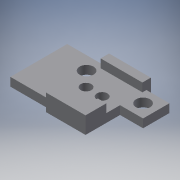
# Autodesk Inventor part: SensorMount
Saved by Autodesk Inventor 2018 (Build 220112000, 112)
## iProperties
Created: 2018-05-09
Part Number: SensorMount
Material: Generic
Document SubType Name: Modeling
Designer: s4321966
Mass: 0.644529 g
Surface Area: 8.91891 cm^2
Volume: 0.644529 cm^3
Density: 1 g/cm^3
Appearance: Default
Author: s4321966
Autodesk Inventor part; units mm, degrees
ref_plane "YZ Plane" through (0, 0, 0) normal (1, 0, 0) x (0, 1, 0)
ref_plane "XZ Plane" through (0, 0, 0) normal (0, 1, 0) x (-1, 0, 0)
ref_plane "XY Plane" through (0, 0, 0) normal (0, 0, 1) x (1, 0, 0)
sketch "Sketch1" plane through (0, 0, 0) normal (0, 0, 1) x (1, 0, 0)
  line L0 (0, 0) -> (15.75, 0)
  line L1 (15.75, 0) -> (15.75, -11.43)
  line L2 (15.75, -11.43) -> (0, -11.43)
  line L3 (0, -11.43) -> (0, 0)
  line L4 (17.75, 2) -> (-2, 2)
  line L5 (-2, 2) -> (-2, -13.43)
  line L6 (-2, -13.43) -> (17.75, -13.43)
  line L7 (17.75, -13.43) -> (17.75, 2)
  dimension "d0" = 15.75
  dimension "d1" = 11.43
  dimension "d2" = 2
  constraints: 16 end point, 4 parallel, 2 perpendicular, 1 horizontal, 3 other
  measures "d0" distance of L1.end L2.end
  measures "d1" distance of L0.end L1.end
  measures "d2" distance between parallel lines of L0 L4
extrude "Extrusion1" add sketch "Sketch1" along normal blind 2
sketch "Sketch2" plane through (0, 0, 0) normal (0, 0, -1) x (-1, 0, 0)
  line L0 (-17.75, 2) -> (2, 2) projected
  line L1 (2, -13.43) -> (-17.75, -13.43) projected
  line L2 (2, 2) -> (-17.75, 2)
  line L3 (-17.75, 2) -> (-17.75, -13.43)
  line L4 (-17.75, -13.43) -> (2, -13.43)
  line L5 (2, -13.43) -> (2, 2)
  point P0 (0, 0)
  constraints: 8 end point, 2 parallel, 1 horizontal, 1 perpendicular
extrude "Extrusion2" add sketch "Sketch2" along normal blind 2
sketch "Sketch3" plane through (0, 0, 0) normal (0, 0, 1) x (1, 0, 0)
  line L0 (0, 0) -> (15.75, 0) projected
  line L1 (0, 0) -> (6.73, 0)
  line L2 (0, 0) -> (6.73, 0) construction
  line L3 (6.73, 0) -> (6.73, -2.16)
  line L4 (15.75, 0) -> (13.84, 0)
  line L5 (15.75, 0) -> (17.66, 0) construction
  line L6 (13.84, 0) -> (13.84, -5.59)
  line L7 (13.84, -5.59) -> (10.04, -5.59)
  circle A0 centre (6.73, -2.16) radius 1.651
  circle A1 centre (10.04, -5.59) radius 1.25
  circle A2 centre (13.84, -5.59) radius 1.25
  dimension "d7" = 6.73
  dimension "d8" = 0
  dimension "d9" = 2.16
  dimension "d10" = 90
  dimension "d11" = 1.91
  dimension "d12" = 180
  dimension "d13" = 5.59
  dimension "d14" = 90
  dimension "d15" = 3.8
  dimension "d16" = 90
  dimension "d17" = 3.302
  dimension "d18" = 2.5
  dimension "d19" = 2.5
  constraints: 14 end point, 3 centre point, 3 coincident, 3 collinear, 3 horizontal, 3 perpendicular
  measures "d7" distance of L0.start L1.end
  measures "d8" distance between parallel lines of L1 L2
  measures "d9" distance of L1.end L3.end
  measures "d10" angle of L1 L3
  measures "d11" distance of L0.end L4.end
  measures "d12" angle of L4 L5
  measures "d13" distance of L4.end L6.end
  measures "d14" angle of L6 L4
  measures "d15" distance of L6.end L7.end
  measures "d16" angle of L6 L7
  measures "d17" diameter of A0
  measures "d18" diameter of A1
  measures "d19" diameter of A2
extrude "Extrusion3" cut sketch "Sketch3" against normal blind 2
sketch "Sketch4" plane through (0, 0, 0) normal (0, 0, 1) x (1, 0, 0)
  circle A0 centre (6.73, -2.16) radius 1.651 projected
  line L0 (6.73, -2.16) -> (-3.27, -2.16)
  circle A1 centre (-3.27, -2.16) radius 1.651
  line L1 (-2, 2) -> (17.75, 2) projected
  line L2 (7.875, 2) -> (-2, 2)
  line L3 (-2, 2) -> (-2, 0)
  line L4 (-2, 0) -> (7.875, 0)
  line L5 (7.875, 0) -> (7.875, 2)
  line L6 (0, -11.43) -> (15.75, -11.43) projected
  line L7 (-2, -13.43) -> (-2, 2) projected
  line L8 (8.381, -11.43) -> (-2, -11.43)
  line L9 (-2, -11.43) -> (-2, -13.43)
  line L10 (-2, -13.43) -> (8.381, -13.43)
  line L11 (8.381, -13.43) -> (8.381, -11.43)
  line L12 (15.75, 0) -> (0, 0) projected
  line L13 (0, 0) -> (-3.27, 0)
  line L14 (-3.27, 0) -> (-3.27, -0.509)
  line L15 (-3.27, -0.509) -> (0, -0.509)
  line L16 (0, -0.509) -> (0, 0)
  line L17 (0, 0) -> (-2, 0)
  line L18 (-2, 0) -> (-2, -11.43)
  line L19 (-2, -11.43) -> (0, -11.43)
  line L20 (0, -11.43) -> (0, 0)
  dimension "d23" = 3.302
  dimension "d22" = 10
  constraints: 34 end point, 8 parallel, 5 horizontal, 4 perpendicular, 1 coincident, 1 midpoint, 1 point on line, 1 vertical alignment, 2 other
  measures "d22" distance of L0.start L0.end
extrude "Extrusion4" cut sketch "Sketch4" along normal mid plane 4 contours L20 L8 L7 A1 L0 | L0 A1 L7 L15 L20 | A1 L7 L0 | L0 L7 A1 | L6 L11 L10 L7 L8 | L15 L7 L4 L16 | L7 A1 | L4 L3 L1 L5
sketch "Sketch5" plane through (0, 0, 0) normal (0, 0, 1) x (1, 0, 0)
  line L0 (15.7294, 0) -> (23.6467, -7.9173)
  line L1 (15.7294, 0) -> (26.9261, 0) construction
  circle A0 centre (13.84, -5.59) radius 1.25 projected
  line L2 (15.09, -5.59) -> (32.9108, -5.59)
  line L3 (32.9108, -5.59) -> (21.3194, -5.59)
  line L4 (21.3194, 0) -> (21.3194, -5.59)
  line L5 (21.3194, -2.795) -> (18.5244, -2.795)
  circle A1 centre (18.5244, -2.795) radius 1.651
  circle A2 centre (6.73, -2.16) radius 1.651 projected
  line L6 (6.73, -2.16) -> (27.3666, -2.16)
  line L7 (18.5244, -2.795) -> (18.5244, 1.4805)
  circle A3 centre (18.5244, -2.16) radius 1.65
  line L8 (17.75, 2) -> (17.75, -13.43) projected
  line L9 (21.3194, 0) -> (17.75, 0)
  line L10 (17.75, 0) -> (17.75, -5.59)
  line L11 (17.75, -5.59) -> (21.3194, -5.59)
  line L12 (21.3194, -5.59) -> (21.3194, 0)
  point P0 (0, 0)
  dimension "d26" = 45
  dimension "d27" = 3.302
  dimension "d28" = 3.3
  constraints: 24 end point, 9 point on line, 5 horizontal, 2 centre point, 2 parallel, 1 coincident, 1 equal length, 1 horizontal alignment, 1 midpoint, 1 perpendicular, 1 vertical, 1 other
  measures "d26" angle of L0 L1
  measures "d27" diameter of A1
  measures "d28" diameter of A3
extrude "Extrusion5" add sketch "Sketch5" against normal blind 2 contours L8 L9 L7 A3 | A3 L7 A1 L8 | L8 A1 L7 L6 L0 | L0 L6 L8 | A3 L6 A1 L7 | L7 L9 L4 L6 A3 | L6 L7 L0 | L0 A3 L8 L6 | A1 L6 L7 | A3 A1 L6 | L6 L4 L5 A1 A3 | L8 A3 L0 A1 | A1 L0 L2 L8 | L5 A3 L0 | L7 L6 A1 A3 L5 | A1 L5 A3 | A1 L5 L4 L0 | L0 A3 L5 A1 picked at (20.1034, -2.1943) picked at (18.7532, -3.9974)
sketch "Sketch6" plane through (0, 0, 2) normal (0, 0, 1) x (1, 0, 0)
  line L0 (21.3194, -5.59) -> (17.75, -5.59) projected
  line L1 (15.75, 0) -> (7.875, 0) projected
  line L2 (17.75, -5.59) -> (15.75, -5.59)
  line L3 (15.75, -5.59) -> (15.75, 0)
  line L4 (15.75, 0) -> (17.75, 0)
  line L5 (17.75, 0) -> (17.75, -5.59)
  line L6 (15.75, -5.59) -> (17.75, -5.59)
  line L7 (17.75, -5.59) -> (17.75, -11.43)
  line L8 (17.75, -11.43) -> (15.75, -11.43)
  line L9 (15.75, -11.43) -> (15.75, -5.59)
  line L10 (15.75, -11.43) -> (15.75, 0) projected
  line L11 (15.75, -8.51) -> (17.75, -8.51)
  line L12 (17.75, -8.51) -> (17.75, -11.43)
  line L13 (17.75, -11.43) -> (15.75, -11.43)
  line L14 (15.75, -11.43) -> (15.75, -8.51)
  point P0 (0, 0)
  constraints: 24 end point, 6 parallel, 3 horizontal, 3 perpendicular, 2 point on line
extrude "Extrusion6" cut sketch "Sketch6" against normal blind 2 contours L7 L11 L9 L2 | L2 L3 L4 L5
sketch "Sketch7" plane through (0, 0, 0) normal (0, 0, 1) x (1, 0, 0)
  circle A0 centre (6.73, -2.16) radius 1.651 projected
  line L0 (6.73, -2.16) -> (25.5258, -2.16)
  line L1 (6.7656, -0.5094) -> (22.9068, -0.5094)
  line L2 (21.3194, 0) -> (17.75, 0) projected
  circle A1 centre (21.3194, 0) radius 0.5094
  line L3 (20.81, 0) -> (20.81, -6.6139)
  line L4 (20.81, -0.5094) -> (15.4003, -5.9192)
  line L5 (20.81, -0.5094) -> (28.4606, -0.5094) construction
  circle A2 centre (19.1594, -2.16) radius 1.651
  point P0 (0, 0)
  dimension "d33" = 135
  dimension "d34" = 3.302
  constraints: 10 end point, 5 point on line, 3 horizontal, 1 centre point, 1 equal length, 1 horizontal alignment, 1 perpendicular, 1 vertical, 4 other
  measures "d33" angle of L4 L5
  measures "d34" diameter of A2
extrude "Extrusion7" cut sketch "Sketch7" against normal blind 2 contours A2 L4 L0 | L0 L4 A2 | L4 A2 L0 | L0 A2 L4
sketch "Sketch8" plane through (0, 0, 0) normal (0, 0, 1) x (1, 0, 0)
  line L0 (15.75, -11.43) -> (15.75, -8.51) projected
  line L1 (15.75, -8.51) -> (15.75, 8.3599)
  line L2 (7.875, 2) -> (17.75, 2) projected
  line L3 (15.75, 2) -> (25.7478, 2) construction
  line L4 (17.75, 0) -> (7.875, 0) projected
  line L5 (15.75, 0) -> (86.4607, -70.7107)
  line L6 (15.75, 0) -> (115.75, 0) construction
  circle A0 centre (6.73, -2.16) radius 1.651 projected
  line L7 (8.381, -2.16) -> (21.8585, -2.16)
  circle A1 centre (17.91, -2.16) radius 1.651
  circle A2 centre (17.91, -2.16) radius 4.1631
  line L8 (15.75, 2) -> (17.91, 2)
  line L9 (17.91, 2) -> (17.91, -6.3231)
  line L10 (17.91, -6.3231) -> (15.75, -6.3231)
  line L11 (15.75, -6.3231) -> (15.75, 2)
  line L12 (17.91, -6.3231) -> (22.0731, -6.3231)
  line L13 (22.0731, -6.3231) -> (22.0731, -2.1615)
  line L14 (22.0731, -2.1615) -> (17.91, -2.1615)
  line L15 (17.91, -2.1615) -> (17.91, -6.3231)
  line L16 (17.91, 2) -> (22.0731, 2)
  line L17 (22.0731, 2) -> (22.0731, -2.1615)
  line L18 (22.0731, -2.1615) -> (17.91, -2.1615)
  line L19 (17.91, -2.1615) -> (17.91, 2)
  point P0 (0, 0)
  dimension "d38" = 100
  dimension "d39" = 45
  dimension "d40" = 3.302
  constraints: 34 end point, 6 horizontal, 6 parallel, 6 point on line, 3 perpendicular, 2 centre point, 2 point on circle, 1 coincident, 1 equal length, 1 horizontal alignment, 1 vertical, 1 other
  measures "d38" distance of L5.start L5.end
  measures "d39" angle of L5 L6
  measures "d40" diameter of A1
extrude "Extrusion8" add sketch "Sketch8" against normal blind 2 contours L1 A2 L10 | A2 L7 L1 | L1 L7 A1 L9 A2 | L9 A1 L5 A2 | A2 L5 L12 | L7 A2 L4 L1 | L1 L5 A1 L7 | A2 L13 L5 | L5 A1 L7 L14 A2 | L9 L5 A1 | A1 L7 L9 | L4 A2 L1 | L1 A2 L8 L9 A1 L5 | A1 L5 L7 | L5 L7 A1 | L14 L7 A1 L9 L16 A2 | A2 L16 L17 | L9 A1 L7 | L5 A1 L9 | L1 L2 A2 | L16 L8 A2
sketch "Sketch9" plane through (0, 0, 0) normal (0, 0, 1) x (1, 0, 0)
  line L0 (17.75, -8.51) -> (15.75, -8.51) projected
  line L1 (15.75, -8.51) -> (15.75, 2.0527)
  line L2 (7.875, 0) -> (17.75, 0) projected
  line L3 (17.75, -6.3231) -> (22.0731, -6.3231) projected
  line L4 (15.75, 0) -> (22.0731, -6.3231)
  circle A0 centre (6.73, -2.16) radius 1.651 projected
  line L5 (6.73, -2.16) -> (23.125, -2.16)
  circle A1 centre (17.91, -2.16) radius 2.16
  point P0 (0, 0)
  constraints: 6 end point, 4 point on line, 1 centre point, 1 horizontal, 1 vertical
extrude "Extrusion9" cut sketch "Sketch9" against normal blind 2 contours A1 L4 L5 | L5 L4 A1 | L5 A1 L4 | L4 A1 L5
sketch "Sketch10" plane through (0, 0, 0) normal (0, 0, 1) x (1, 0, 0)
  line L0 (15.75, -11.43) -> (15.75, -8.51) projected
  line L1 (0, 0) -> (15.75, 0)
  line L2 (15.75, 0) -> (15.75, -11.43)
  line L3 (15.75, -11.43) -> (0, -11.43)
  line L4 (0, -11.43) -> (0, 0)
  line L5 (-1, -12.43) -> (16.75, -12.43)
  line L6 (16.75, -12.43) -> (16.75, 1)
  line L7 (16.75, 1) -> (-1, 1)
  line L8 (-1, 1) -> (-1, -12.43)
  circle A0 centre (17.91, -2.16) radius 2.16 projected
  circle A1 centre (17.91, -2.16) radius 2.16
  line L9 (8.381, -13.43) -> (8.381, -11.43) projected
  line L10 (8.381, -12.43) -> (-1, -12.43)
  line L11 (-1, -12.43) -> (-1, -11.43)
  line L12 (-1, -11.43) -> (8.381, -11.43)
  line L13 (8.381, -11.43) -> (8.381, -12.43)
  line L14 (-1, -11.43) -> (0, -11.43)
  line L15 (0, -11.43) -> (0, 1)
  line L16 (0, 1) -> (-1, 1)
  line L17 (-1, 1) -> (-1, -11.43)
  line L18 (7.875, 0) -> (7.875, 2) projected
  line L19 (7.875, 0) -> (0, 0)
  line L20 (0, 0) -> (0, 1)
  line L21 (0, 1) -> (7.875, 1)
  line L22 (7.875, 1) -> (7.875, 0)
  dimension "d45" = 1
  constraints: 40 end point, 10 parallel, 5 perpendicular, 4 horizontal, 2 point on line, 1 centre point, 1 coincident, 1 midpoint, 3 other
  measures "d45" distance between parallel lines of L3 L5
extrude "Extrusion10" add sketch "Sketch10" against normal blind 2 contours L9 L5 L8 L12 L3 | L12 L8 L7 L15 L4 | L15 L7 L18 L1
sketch "Sketch11" plane through (0, 0, 0) normal (0, 0, 1) x (1, 0, 0)
  line L0 (6.1748, 0.9529) -> (26.8084, 0.9529)
  circle A0 centre (17.91, -2.16) radius 2.16 projected
  circle A1 centre (17.91, -2.16) radius 3.164
  line L1 (17.75, -6.3231) -> (17.75, -8.51) projected
  line L2 (22.0731, -6.3231) -> (22.0731, 2) projected
  line L3 (17.75, -6.3231) -> (22.0731, -6.3231)
  line L4 (22.0731, -6.3231) -> (22.0731, -5.324)
  line L5 (22.0731, -5.324) -> (17.75, -5.324)
  line L6 (17.75, -5.324) -> (17.75, -6.3231)
  line L7 (22.0731, -5.324) -> (21.074, -5.324)
  line L8 (21.074, -5.324) -> (21.074, 0.9529)
  line L9 (21.074, 0.9529) -> (22.0731, 0.9529)
  line L10 (22.0731, 0.9529) -> (22.0731, -5.324)
  line L11 (17.75, 0) -> (17.75, 2) projected
  line L12 (17.75, 2) -> (22.0731, 2)
  line L13 (22.0731, 2) -> (22.0731, 0.9529)
  line L14 (22.0731, 0.9529) -> (17.75, 0.9529)
  line L15 (17.75, 0.9529) -> (17.75, 2)
  line L16 (17.75, 1.7899) -> (23.3786, 1.7899)
  line L17 (23.3786, 1.7899) -> (23.3786, 10.3517)
  line L18 (23.3786, 10.3517) -> (17.75, 10.3517)
  line L19 (17.75, 10.3517) -> (17.75, 1.7899)
  line L20 (17.75, -6.0225) -> (23.2057, -6.0225)
  line L21 (23.2057, -6.0225) -> (23.2057, -7.1179)
  line L22 (23.2057, -7.1179) -> (17.75, -7.1179)
  line L23 (17.75, -7.1179) -> (17.75, -6.0225)
  line L24 (21.5736, -6.5702) -> (23.2057, -6.5702)
  line L25 (23.2057, -6.5702) -> (23.2057, 4.5573)
  line L26 (23.2057, 4.5573) -> (21.5736, 4.5573)
  line L27 (21.5736, 4.5573) -> (21.5736, -6.5702)
  point P0 (0, 0)
  constraints: 50 end point, 12 parallel, 7 horizontal, 6 perpendicular, 5 point on line, 1 centre point, 1 coincident
extrude "Extrusion11" cut sketch "Sketch11" against normal blind 2 contours L11 A1 L0 | L11 L16 L27 L0 A1 | L5 L27 L20 L6 | L11 L12 L27 L16 | L8 L0 L27 L5 | L19 L18 L17 L16 L25 L26 L27 L12 | L27 L12 L2 L16 | L16 L2 L0 L27 | L27 L0 L2 L5 | L5 L2 L20 L27 | L20 L27 L3 L6 | L27 L26 L25 L16 L2 L12 | L16 L25 L0 L2 | L2 L0 L25 L20 | L20 L2 L3 L27 | L3 L27 L24 L21 L22 L1 | L20 L21 L24 L27 L3 L2 picked at (18.154, 0.9643)
sketch "Sketch12" plane through (0, 0, 0) normal (0, 0, 1) x (1, 0, 0)
  arc A0 (14.4765, -4.5142) -> (15.0081, -5.145) centre (13.84, -5.59) ccw projected
  circle A1 centre (13.84, -5.59) radius 1.25
  circle A2 centre (17.91, -2.16) radius 2.16 projected
  circle A3 centre (20.07, -2.16) radius 2.16
  point P0 (0, 0)
  constraints: 2 horizontal alignment, 1 centre point, 1 coincident, 3 other
extrude "Extrusion12" cut sketch "Sketch12" against normal blind 2
sketch "Sketch13" plane through (0, 0, 0) normal (0, 0, 1) x (1, 0, 0)
  arc A0 (21.074, -0.2475) -> (18.99, -0.2894) centre (20.07, -2.16) ccw projected
  circle A1 centre (20.07, -2.16) radius 2.16
  line L0 (20.07, 0) -> (16.3795, 0.6879)
  line L1 (16.3795, 0.6879) -> (14.9709, -1.081)
  line L2 (14.9709, -1.081) -> (14.9709, -3.5052)
  line L3 (14.9709, -3.5052) -> (15.3588, -4.788)
  line L4 (15.3588, -4.788) -> (16.6942, -5.0369)
  line L5 (16.6942, -5.0369) -> (18.99, -4.788)
  line L6 (18.99, -4.788) -> (18.99, -4.0306)
  point P0 (0, 0)
  constraints: 14 end point, 3 point on circle, 1 centre point, 1 coincident, 1 parallel, 1 vertical
extrude "Extrusion13" add sketch "Sketch13" against normal blind 2 contours A0 A1 L6 L5 L4 L3 L2 L1 L0
sketch "Sketch14" plane through (0, 0, 0) normal (0, 0, 1) x (1, 0, 0)
  arc A0 (21.074, -0.2475) -> (21.074, -4.0725) centre (20.07, -2.16) ccw projected
  circle A1 centre (20.07, -2.16) radius 2.16
  circle A2 centre (20.07, -2.16) radius 3.1129
  line L0 (21.074, 0.9529) -> (17.75, 0.9529) projected
  line L1 (20.07, -2.16) -> (23.1829, -2.16)
  line L2 (23.1829, -2.16) -> (23.1829, 0.9529)
  line L3 (23.1829, 0.9529) -> (20.07, 0.9529)
  line L4 (20.07, 0.9529) -> (20.07, -2.16)
  line L5 (17.75, -5.324) -> (21.074, -5.324) projected
  line L6 (23.1829, -2.16) -> (20.07, -2.16)
  line L7 (20.07, -2.16) -> (20.07, -5.324)
  line L8 (20.07, -5.324) -> (23.1829, -5.324)
  line L9 (23.1829, -5.324) -> (23.1829, -2.16)
  point P0 (0, 0)
  constraints: 16 end point, 4 parallel, 2 centre point, 2 coincident, 2 horizontal, 2 perpendicular, 2 point on line, 1 tangent
extrude "Extrusion14" add sketch "Sketch14" against normal blind 2 contours A0 L4 A2 L1 A1 | A0 L7 A2 L4 | L1 A2 L7 A0 A1
sketch "Sketch15" plane through (0, 0, 0) normal (0, 0, 1) x (1, 0, 0)
  arc A0 (21.074, -5.1065) -> (21.074, 0.7865) centre (20.07, -2.16) ccw projected
  line L0 (17.75, 0.9529) -> (21.074, 0.9529) projected
  line L1 (23.1829, -2.16) -> (20.1705, -2.16)
  line L2 (20.1705, 0.9529) -> (23.1829, 0.9529)
  line L3 (23.1829, 0.9529) -> (23.1829, -2.16)
  line L4 (23.1829, -2.16) -> (20.07, -2.16)
  line L5 (20.07, -5.2729) -> (23.1829, -5.2729)
  line L6 (23.1829, -5.2729) -> (23.1829, -2.16)
  circle A1 centre (20.07, -2.16) radius 2.16 projected
  arc A2 (20.07, -4.32) -> (20.1705, -0.0023) centre (20.07, -2.16) ccw
  line L7 (20.1705, 0.9529) -> (20.1705, -0.0023)
  line L8 (20.07, -4.32) -> (20.07, -5.2729)
  line L9 (21.074, -5.324) -> (17.75, -5.324) projected
  point P0 (0, 0)
  constraints: 16 end point, 5 point on circle, 2 horizontal, 2 parallel, 1 centre point, 1 perpendicular, 1 point on line, 1 vertical
extrude "Extrusion15" add sketch "Sketch15" against normal blind 2 contours L0 L2 L3 L1 A1 L7 | L1 L6 L5 L8 A1
sketch "Sketch16" plane through (0, 0, 0) normal (0, 0, 1) x (1, 0, 0)
  circle A0 centre (20.07, -2.16) radius 2.16 projected
  circle A1 centre (20.07, -2.16) radius 3.1129
  line L0 (23.1829, 0.9529) -> (17.75, 0.9529) projected
  line L1 (20.07, -5.2729) -> (23.1829, -5.2729)
  line L2 (23.1829, -5.2729) -> (23.1829, -5.4822)
  line L3 (23.1829, -5.4822) -> (20.07, -5.4822)
  line L4 (20.07, -5.4822) -> (20.07, -5.2729)
  line L5 (20.07, -5.2729) -> (17.75, -5.2729)
  line L6 (17.75, -5.2729) -> (17.75, -5.5501)
  line L7 (17.75, -5.5501) -> (20.07, -5.5501)
  line L8 (20.07, -5.5501) -> (20.07, -5.2729)
  point P0 (0, 0)
  constraints: 16 end point, 4 parallel, 3 horizontal, 2 perpendicular, 1 coincident, 1 vertical alignment, 2 other
extrude "Extrusion16" cut sketch "Sketch16" against normal blind 2 contours L1 L2 L3 L4 | L4 L8 L7 L6 L5
sketch "Sketch17" plane through (0, 0, 0) normal (0, 0, 1) x (1, 0, 0)
  circle A0 centre (20.07, -2.16) radius 2.16 projected
  circle A1 centre (20.07, -2.16) radius 2.16
  circle A2 centre (20.07, -2.16) radius 1.651
  point P0 (0, 0)
  dimension "d60" = 3.302
  constraints: 2 centre point, 2 coincident
  measures "d60" diameter of A2
extrude "Extrusion17" add sketch "Sketch17" against normal blind 2
body "Solid1"
